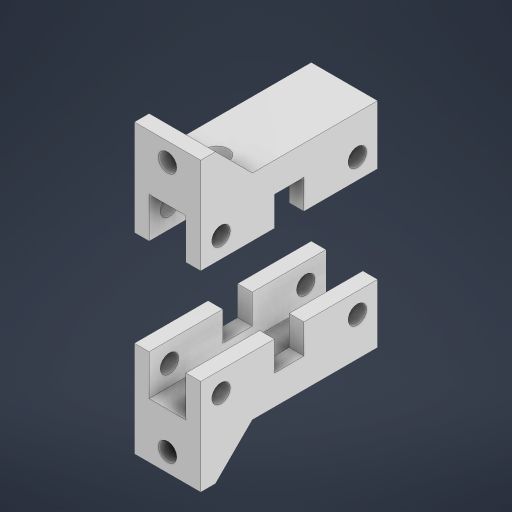
# Autodesk Inventor part: 2020_guide_adaptor
Saved by Autodesk Inventor 2024 (Build 280153000, 153)
## iProperties
Created: 2026-03-27
Part Number: 2020_guide_adaptor
Material: PET Plastic
Document SubType Name: Modeling
Designer: schar
Density: 1.541 g/cm^3
Appearance: Polycarbonate - Clear
Author: schar
Autodesk Inventor part; units mm, degrees
ref_plane "YZ Plane" through (0, 0, 0) normal (1, 0, 0) x (0, 1, 0)
ref_plane "XZ Plane" through (0, 0, 0) normal (0, 1, 0) x (-1, 0, 0)
ref_plane "XY Plane" through (0, 0, 0) normal (0, 0, 1) x (1, 0, 0)
sketch "Sketch3" plane through (0, 0, 0) normal (0, 0, 1) x (1, 0, 0)
  line L0 (-0.0001, 48.0001) -> (-10.0001, 48.0001)
  line L1 (-0.0001, 42.5001) -> (-0.0001, 48.0001)
  line L2 (-0.0001, 5.5001) -> (-0.0001, 42.5001)
  line L3 (-0.0001, 0) -> (-0.0001, 5.5001)
  line L4 (-10, 3) -> (0, 3)
  line L5 (-10.0001, 5.5001) -> (-10.0001, 42.5001)
  line L6 (-10.0001, 5.5001) -> (-10.0001, 0.0001)
  line L7 (-10.0001, 48.0001) -> (-10.0001, 42.5001)
  line L8 (-0.0001, 48.0001) -> (-10, 48.0001)
  line L9 (-10, 48.0001) -> (-10, 53.0001)
  line L10 (-10, 53.0001) -> (-0.0001, 53.0001)
  line L11 (-0.0001, 53.0001) -> (-0.0001, 48.0001)
  line L12 (-10, 3) -> (0, 3)
  line L13 (0, 3) -> (0, -2)
  line L14 (0, -2) -> (-10, -2)
  line L15 (-10, -2) -> (-10, 3)
  line L16 (-10, 53.0001) -> (-14, 53.0001)
  line L17 (-14, 53.0001) -> (-14, 37.0001)
  line L18 (-14, 37.0001) -> (-10, 37.0001)
  line L19 (-10, 37.0001) -> (-10, 53.0001)
  line L20 (0, 24) -> (-10, 24)
  line L21 (-0.0001, 53.0001) -> (3.9999, 53.0001)
  line L22 (3.9999, 53.0001) -> (3.9999, 37.0001)
  line L23 (3.9999, 37.0001) -> (-0.0001, 37.0001)
  line L24 (-0.0001, 37.0001) -> (-0.0001, 53.0001)
  line L25 (0, 0) -> (-10.0001, -0.0001)
  line L26 (-0.0001, 5.5001) -> (0, 0)
  line L27 (-10.0001, -0.0001) -> (-10.0001, 5.5001)
  line L28 (0, 0) -> (-10, -0.0001)
  line L29 (-10, -0.0001) -> (-10, -5.0001)
  line L30 (-10, -5.0001) -> (-0.0001, -5.0001)
  line L31 (-0.0001, -5.0001) -> (0, 0)
  line L32 (-10, -5.0001) -> (-14, -5.0001)
  line L33 (-14, -5.0001) -> (-14, 10.9999)
  line L34 (-14, 10.9999) -> (-10, 10.9999)
  line L35 (-10, 10.9999) -> (-10, -5.0001)
  line L36 (-0.0001, -5.0001) -> (3.9999, -5.0001)
  line L37 (3.9999, -5.0001) -> (3.9999, 10.9999)
  line L38 (3.9999, 10.9999) -> (-0.0001, 10.9999)
  line L39 (-0.0001, 10.9999) -> (-0.0001, -5.0001)
  point P0 (-10.0001, 0.0001)
  point P1 (-0.0001, 10.9999)
  point P2 (-10, 0)
  point P3 (-10.0001, 10.9999)
  point P4 (-10.0001, 37.0001)
  point P5 (-0.0001, 37.0001)
  point P6 (-0.0001, 0)
  point P7 (-10.0001, 0.0001)
  point P8 (-10, -0.0001)
extrude "Extrusion1" add sketch "Sketch3" against normal blind 48 contours L11 L21 L22 L23 L2 L1 | L0 L9 L10 L11 | L7 L5 L18 L17 L16 L9 | L38 L37 L36 L31 L13 L3 L2 | L5 L6 L15 L29 L32 L33 L34 | L13 L14 L15 L25 | L30 L29 L14 L31
sketch "Sketch4" plane through (3.9999, -5.0001, 0) normal (1, 0, 0) x (0, 0, -1)
  line L0 (22, 27.0002) -> (22, 10.0002) projected
  line L1 (26, 27.0002) -> (26, 10.0002) projected
  circle A0 centre (5.5, 10.5002) radius 2.5 projected
  circle A1 centre (42.5, 10.5002) radius 2.5 projected
  line L2 (22, 10) -> (26, 10) projected
  line L3 (-9.6, 29) -> (57.6, 29)
  line L4 (-9.6, 29) -> (57.6, 29)
  line L5 (22, 16.019) -> (20, 16.019)
  line L6 (20, 16.019) -> (20, 8.019)
  line L7 (26, 16.019) -> (28, 16.019)
  line L8 (28, 16.019) -> (28, 8.019)
  line L9 (28, 8.019) -> (20, 8.019)
  line L10 (20, 16.019) -> (28, 16.019)
  circle A2 centre (5.5, 47.4998) radius 2.5
  circle A3 centre (42.5, 47.4998) radius 2.5
  line L11 (20, 41.981) -> (20, 49.981)
  line L12 (28, 41.981) -> (28, 49.981)
  line L13 (28, 49.981) -> (20, 49.981)
  line L14 (20, 41.981) -> (28, 41.981)
  point P0 (0, 5.0001)
  point P1 (26, 41.981)
  dimension "d8" = 2
  dimension "d9" = 8
  dimension "d10" = 2
  constraints: 24 end point, 7 symmetric about line, 5 horizontal, 3 perpendicular, 2 centre point, 2 point on line, 4 other
  measures "d8" distance of L5.start L5.end
  measures "d9" distance of L5.end L6.end
  measures "d10" distance of L7.start L7.end
extrude "Extrusion2" cut sketch "Sketch4" against normal through all
sketch "Sketch5" plane through (0, 0, 0) normal (0, 0, 1) x (1, 0, 0)
  line L0 (3.9999, -5.0001) -> (-14, -5.0001) projected
  line L1 (-103.5812, 24) -> (13.5812, 24)
  line L2 (7.6307, 24) -> (-16.2188, 24)
  line L3 (-5.0001, -5.0001) -> (-5.0001, -15.0001)
  line L4 (-0.0001, -5.0001) -> (-0.0001, -15.0001)
  line L5 (-0.0001, -15.0001) -> (-10.0001, -15.0001)
  line L6 (-10.0001, -15.0001) -> (-10.0001, -5.0001)
  line L7 (-10.0001, -5.0001) -> (-0.0001, -5.0001)
  line L8 (-0.0001, -5.0001) -> (-10.0001, -15.0001) construction
  line L9 (-0.0001, -15.0001) -> (-10.0001, -5.0001) construction
  circle A0 centre (-5.0001, -10.0001) radius 2.5
  line L10 (-0.0001, -15.0001) -> (3.9999, -15.0001)
  line L11 (3.9999, -15.0001) -> (3.9999, -5.0001)
  line L12 (3.9999, -5.0001) -> (-0.0001, -5.0001)
  line L13 (-0.0001, -5.0001) -> (-0.0001, -15.0001)
  line L14 (-10.0001, -15.0001) -> (-14, -15.0001)
  line L15 (-14, -15.0001) -> (-14, -5.0001)
  line L16 (-14, -5.0001) -> (-10.0001, -5.0001)
  line L17 (-10.0001, -5.0001) -> (-10.0001, -15.0001)
  line L18 (3.9999, 53.0001) -> (-14, 53.0001)
  line L19 (-5.0001, 53.0001) -> (-5.0001, 63.0001)
  line L20 (-0.0001, 53.0001) -> (-0.0001, 63.0001)
  line L21 (-0.0001, 63.0001) -> (-10.0001, 63.0001)
  line L22 (-10.0001, 63.0001) -> (-10.0001, 53.0001)
  line L23 (-10.0001, 53.0001) -> (-0.0001, 53.0001)
  line L24 (-0.0001, 53.0001) -> (-10.0001, 63.0001) construction
  line L25 (-0.0001, 63.0001) -> (-10.0001, 53.0001) construction
  circle A1 centre (-5.0001, 58.0001) radius 2.5
  line L26 (-0.0001, 63.0001) -> (3.9999, 63.0001)
  line L27 (3.9999, 63.0001) -> (3.9999, 53.0001)
  line L28 (3.9999, 53.0001) -> (-0.0001, 53.0001)
  line L29 (-0.0001, 53.0001) -> (-0.0001, 63.0001)
  line L30 (-10.0001, 63.0001) -> (-14, 63.0001)
  line L31 (-14, 63.0001) -> (-14, 53.0001)
  line L32 (-14, 53.0001) -> (-10.0001, 53.0001)
  line L33 (-10.0001, 53.0001) -> (-10.0001, 63.0001)
  point P0 (0, 0)
  dimension "d13" = 10
  dimension "d14" = 10
  dimension "d15" = 5
  constraints: 66 end point, 14 symmetric about line, 6 midpoint, 6 parallel, 3 horizontal, 3 perpendicular, 2 centre point, 2 coincident, 2 point on line, 2 vertical, 3 other
  measures "d13" distance of L3.start L3.end
  measures "d14" distance of L4.end L5.end
  measures "d15" diameter of A0
extrude "Extrusion3" add sketch "Sketch5" against normal blind 4 contours L11 L10 L4 L0 | L4 L5 L3 A0 L0 | L3 A0 L5 L6 L0 | L6 L14 L15 L0 | L18 L20 L26 L27 | L18 L19 A1 L21 L20 | L18 L22 L21 L19 A1 | L18 L31 L30 L22
sketch "Sketch6" plane through (0, 0, -4) normal (0, 0, -1) x (-1, 0, 0)
  line L0 (-3.9999, -5.0001) -> (-3.9999, -15.0001) projected
  line L1 (-3.9999, -15.0001) -> (0.0001, -15.0001)
  line L2 (0.0001, -15.0001) -> (0.0001, -5.0001)
  line L3 (0.0001, -5.0001) -> (-3.9999, -5.0001)
  line L4 (-3.9999, -5.0001) -> (-3.9999, -15.0001)
  line L5 (14, 10.9999) -> (14, -15.0001) projected
  line L6 (14, -5.0001) -> (10, -5.0001)
  line L7 (10, -5.0001) -> (10, -15.0001)
  line L8 (10, -15.0001) -> (14, -15.0001)
  line L9 (14, -15.0001) -> (14, -5.0001)
  line L10 (-13.5812, 24) -> (103.5812, 24)
  line L11 (-3.9999, 53.0001) -> (-3.9999, 63.0001)
  line L12 (-3.9999, 63.0001) -> (0.0001, 63.0001)
  line L13 (0.0001, 63.0001) -> (0.0001, 53.0001)
  line L14 (0.0001, 53.0001) -> (-3.9999, 53.0001)
  line L15 (14, 37.0001) -> (14, 63.0001)
  line L16 (14, 53.0001) -> (10, 53.0001)
  line L17 (10, 53.0001) -> (10, 63.0001)
  line L18 (10, 63.0001) -> (14, 63.0001)
  point P0 (0, 0)
  point P1 (-3.9999, -5.0001)
  dimension "d18" = 4
  constraints: 34 end point, 11 symmetric about line, 6 point on line, 4 parallel, 3 horizontal, 2 perpendicular, 2 other
  measures "d18" distance of L8.end L7.end
extrude "Extrusion4" add sketch "Sketch6" along normal blind 10
sketch "Sketch7" plane through (3.9999, -5.0001, -48) normal (1, 0, 0) x (0, 0, -1)
  line L0 (-48, -10) -> (-34, -10) projected
  line L1 (-34, -10) -> (-44, -10)
  line L2 (-34, 0) -> (0, 0) projected
  line L3 (-44, -10) -> (-34, 0)
  line L4 (-34, 0) -> (-34, -10) projected
  line L5 (-34, -10) -> (-34, 0)
  line L6 (-34, 68.0002) -> (-34, 58.0002) projected
  line L7 (-34, 58.0002) -> (-34, 68.0002)
  line L8 (-34, 68.0002) -> (-44, 68.0002)
  line L9 (-44, 68.0002) -> (-34, 58.0002)
  point P0 (-48, 5.0001)
  dimension "d21" = 10
  dimension "d22" = 10
  constraints: 12 end point, 1 collinear, 1 perpendicular, 1 point on line, 1 vertical
  measures "d21" distance of L0.end L1.end
  measures "d22" distance of L6.start L8.end
extrude "Extrusion5" cut sketch "Sketch7" against normal through all
sketch "Sketch8" plane through (-14, -5.0001, -48) normal (0, -1, 0) x (1, 0, 0)
  circle A0 centre (8.9999, 34.5) radius 3
  point P0 (14, 48)
  constraints: 1 centre point, 2 other
extrude "Extrusion6" cut sketch "Sketch8" against normal through all
body "Solid1"
